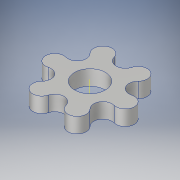
# Autodesk Inventor part: Turret Drive Gear
Saved by Autodesk Inventor 2019.4 (Build 234330000, 330)
## iProperties
Created: 2020-01-12
Part Number: Turret Drive Gear
Material: Aluminum 6061
Document SubType Name: Modeling
Designer: admin
Density: 2.7 g/cm^3
Appearance: Aluminum - Flat
Author: admin
Autodesk Inventor part; units mm, degrees
ref_plane "YZ Plane" through (0, 0, 0) normal (1, 0, 0) x (0, 1, 0)
ref_plane "XZ Plane" through (0, 0, 0) normal (0, 1, 0) x (-1, 0, 0)
ref_plane "XY Plane" through (0, 0, 0) normal (0, 0, 1) x (1, 0, 0)
sketch "Sketch1" plane through (0, 0, 0) normal (0, 1, 0) x (-1, 0, 0)
  circle A0 centre (0, 0) radius 7.3323 construction
  circle A1 centre (0, 0) radius 11.5911 construction
  line L0 (7.3323, 0) -> (3.6662, -6.35)
  line L1 (3.6662, -6.35) -> (-3.6662, -6.35)
  line L2 (-3.6662, -6.35) -> (-7.3323, 0)
  line L3 (-7.3323, 0) -> (-3.6662, 6.35)
  line L4 (-3.6662, 6.35) -> (3.6662, 6.35)
  line L5 (3.6662, 6.35) -> (7.3323, 0)
  arc A2 (10.8147, -2.8978) -> (11.6479, 2.9995) centre (11.5911, 0) ccw
  arc A3 (10.8147, -2.8978) -> (7.9169, -7.9169) centre (10.0382, -5.7956) ccw
  arc A4 (2.8978, -10.8147) -> (7.9169, -7.9169) centre (5.7956, -10.0382) ccw
  arc A5 (2.8978, -10.8147) -> (-2.682, -10.247) centre (0, -11.5911) ccw
  line L6 (11.5911, 0) -> (0, 0) construction
  line L7 (0, 0) -> (5.7956, -10.0382) construction
  line L8 (7.3323, 0) -> (14.5911, 0)
  line L9 (3.6662, -6.35) -> (7.2956, -12.6363)
  dimension "d1" = 3
  dimension "d2" = 3
  dimension "d3" = 3
  dimension "d4" = 3
  dimension "d5" = 60
  dimension "d15" = 12.7
  constraints: 20 end point, 14 point on circle, 5 centre point, 3 coincident, 3 equal radius, 3 horizontal, 1 horizontal alignment, 1 line through centre, 15 other
  measures "d1" radius of A2
  measures "d2" radius of A3
  measures "d3" radius of A4
  measures "d4" radius of A5
  measures "d5" angle of L7 L6
  measures "d15" distance between parallel lines of L4 L1
extrude "Extrusion1" add sketch "Sketch1" along normal blind 5 contours L8 A2 A3 A4 L9 L0
pattern_circular "Circular Pattern1" count 6 over 360 about axis through (0, -10, 0) along (0, 1, 0) of "Extrusion1"
sketch "Sketch3" plane through (0, 5, 0) normal (0, 1, 0) x (1, 0, 0)
  circle A0 centre (0, 0) radius 5.05
  arc A1 (-2.8978, 10.8147) -> (-7.9169, 7.9169) centre (-5.7956, 10.0382) ccw projected
  arc A2 (-10.8147, 2.8978) -> (-7.9169, 7.9169) centre (-10.0382, 5.7956) ccw projected
  arc A3 (-10.8147, 2.8978) -> (-10.8147, -2.8978) centre (-11.5911, 0) ccw projected
  arc A4 (-7.9169, -7.9169) -> (-10.8147, -2.8978) centre (-10.0382, -5.7956) ccw projected
  arc A5 (-7.9169, -7.9169) -> (-2.8978, -10.8147) centre (-5.7956, -10.0382) ccw projected
  arc A6 (2.8978, -10.8147) -> (-2.8978, -10.8147) centre (0, -11.5911) ccw projected
  arc A7 (2.8978, -10.8147) -> (7.9169, -7.9169) centre (5.7956, -10.0382) ccw projected
  arc A8 (10.8147, -2.8978) -> (7.9169, -7.9169) centre (10.0382, -5.7956) ccw projected
  arc A9 (10.8147, -2.8978) -> (10.8147, 2.8978) centre (11.5911, 0) ccw projected
  arc A10 (7.9169, 7.9169) -> (10.8147, 2.8978) centre (10.0382, 5.7956) ccw projected
  arc A11 (7.9169, 7.9169) -> (2.8978, 10.8147) centre (5.7956, 10.0382) ccw projected
  arc A12 (-2.8978, 10.8147) -> (2.8978, 10.8147) centre (0, 11.5911) ccw projected
  line L0 (-3.6662, 6.35) -> (3.6662, 6.35) projected
  line L1 (3.6662, 6.35) -> (7.3323, 0) projected
  line L2 (7.3323, 0) -> (3.6662, -6.35) projected
  line L3 (3.6662, -6.35) -> (-3.6662, -6.35) projected
  line L4 (-3.6662, -6.35) -> (-7.3323, 0) projected
  line L5 (-7.3323, 0) -> (-3.6662, 6.35) projected
  dimension "d16" = 10.1
  constraints: 1 centre point, 1 coincident
  measures "d16" diameter of A0
extrude "Extrusion3" add sketch "Sketch3" against normal up to surface (5 mm away) contours L0 L1 L2 L3 L4 L5
equation "\"d2\" = d1"
equation "\"d3\" = d2"
equation "\"d4\" = d3"
body "Solid1"
